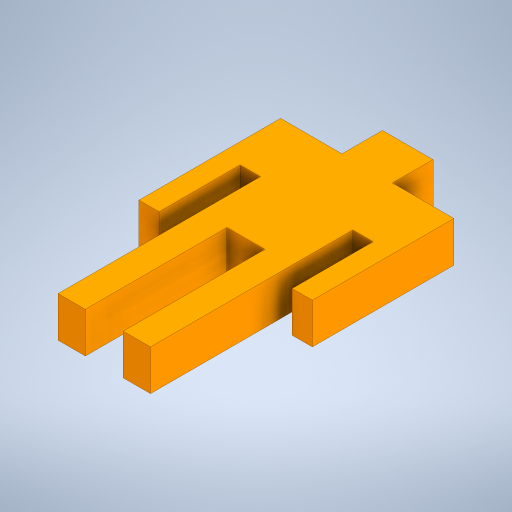
# Autodesk Inventor part: human_model
Saved by Autodesk Inventor 2024.1 (Build 281209000, 209)
## iProperties
Created: 2025-01-27
Part Number: human_model
Material: 一般
Document SubType Name: Modeling
Designer: hibik
Density: 1 g/cm^3
Appearance: 既定
Author: hibik
Autodesk Inventor part; units mm, degrees
ref_plane "YZ Plane" through (0, 0, 0) normal (1, 0, 0) x (0, 1, 0)
ref_plane "XZ Plane" through (0, 0, 0) normal (0, 1, 0) x (-1, 0, 0)
ref_plane "XY Plane" through (0, 0, 0) normal (0, 0, 1) x (1, 0, 0)
sketch "スケッチ1" plane through (0, 0, 0) normal (0, 1, 0) x (-1, 0, 0)
  line L0 (45.7143, 140) -> (25.7143, 140)
  line L1 (25.7143, 140) -> (25.7143, 0)
  line L2 (25.7143, 0) -> (45.7143, 0)
  line L3 (45.7143, 0) -> (45.7143, 140)
  line L4 (45.7143, 0) -> (0, 0)
  line L5 (0, 0) -> (0, -120)
  line L6 (0, -120) -> (45.7143, -120)
  line L7 (45.7143, -120) -> (45.7143, 0)
  line L8 (25, -120) -> (0, -120)
  line L9 (0, -120) -> (0, -160)
  line L10 (0, -160) -> (25, -160)
  line L11 (25, -160) -> (25, -120)
  line L12 (45.7143, -120) -> (65.7143, -120)
  line L13 (65.7143, -120) -> (65.7143, -60)
  line L14 (65.7143, -60) -> (45.7143, -60)
  line L15 (45.7143, -60) -> (45.7143, -120)
  line L16 (65.7143, -120) -> (85.7143, -120)
  line L17 (85.7143, -120) -> (85.7143, 20)
  line L18 (85.7143, 20) -> (65.7143, 20)
  line L19 (65.7143, 20) -> (65.7143, -120)
  line L20 (0, -220) -> (0, 200) projected
  line L21 (102.8571, 0) -> (-17.1429, 0) projected
  line L22 (25.7143, 0) -> (25.7143, 140)
  line L23 (25.7143, 0) -> (18.7143, 0)
  line L24 (18.7143, 0) -> (18.7143, 140)
  line L25 (18.7143, 140) -> (25.7143, 140)
  line L26 (25.7143, 140) -> (25.7143, 0)
  point P0 (0, 0)
  point P1 (65.7143, 0)
  point P2 (25.7143, 0)
  point P3 (18.7143, 0)
  dimension "d0" = 40
  dimension "d2" = 300
  dimension "d3" = 140
  dimension "d4" = 85.7143
  dimension "d5" = 20
  dimension "d6" = 20
  dimension "d7" = 25
  dimension "d10" = 60
  dimension "d11" = 7
  constraints: 50 end point, 14 parallel, 9 collinear, 6 horizontal, 6 perpendicular, 2 point on line
  measures "d0" distance of L10.end L8.start
  measures "d2" distance between parallel lines of L10 L0
  measures "d3" distance of L2.end L0.start
  measures "d4" distance between parallel lines of L20 L17
  measures "d5" distance between parallel lines of L3 L1
  measures "d6" distance between parallel lines of L4 L18
  measures "d7" distance of L9.end L10.end
  measures "d10" distance between parallel lines of L12 L14
  measures "d11" distance between parallel lines of L1 L24
extrude "押し出し1" add sketch "スケッチ1" along normal blind 40 contours L3 L2 L1 L0 | L1 L4 L24 L25 | L7 L6 L5 L4 L2 | L14 L13 L12 L7 | L21 L17 L16 L13 L19 | L19 L18 L17 L21 | L11 L10 L9 L6
mirror "ミラー1" about plane through (0, 0, 0) normal (1, 0, 0)
